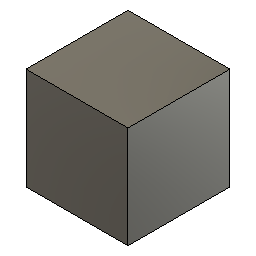
Cube_v1 (Autodesk Fusion 360 design; units mm, degrees)
Autodesk Fusion 360 part; units mm, degrees
box "BoxPrimitive1" add length 35 width 35 height 35 placed x (0, 0, -1) y (-1, 0, 0) z (0, 1, 0) at (35, 0, 0)
